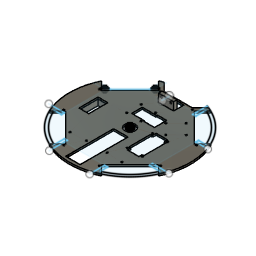
全国オフェンス上面v3 v13 (Autodesk Fusion 360 design; units mm, degrees)
Autodesk Fusion 360 part; units mm, degrees
sketch "スケッチ1" plane through (0, 0, 0) normal (0, 0, 1) x (1, 0, 0)
sketch "スケッチ2" plane through (0, 0, 0) normal (0, 0, 1) x (1, 0, 0)
  line L0 (105, 0) -> (105, 35)
  line L1 (105, 35) -> (98.9949, 35)
  line L2 (98.9949, 35) -> (78.9949, 35)
  line L3 (78.9949, 35) -> (105, 35)
  line L4 (105, 35) -> (105, -35)
  line L5 (105, -35) -> (78.9949, -35)
  line L6 (78.9949, -35) -> (78.9949, 35)
  line L7 (0, 105) -> (35, 105)
  line L8 (35, 105) -> (-35, 105)
  line L9 (-35, 105) -> (-35, 78.995)
  line L10 (-35, 78.995) -> (35, 78.995)
  line L11 (35, 78.995) -> (35, 105)
  line L12 (-105, 0) -> (-105, -35)
  line L13 (-105, -35) -> (-78.995, -35)
  line L14 (-78.995, -35) -> (-78.995, 34.9927)
  line L15 (-78.995, 34.9927) -> (-105, 34.9927)
  line L16 (-105, 34.9927) -> (-105, -35)
  line L17 (0, -105) -> (35, -105)
  line L18 (35, -105) -> (-35, -105)
  line L19 (-35, -105) -> (-35, -78.995)
  line L20 (-35, -78.995) -> (35, -78.995)
  line L21 (35, -78.995) -> (35, -105)
  arc A0 (-98.9949, -35) -> (-35, -98.9949) centre (0, 0) ccw
  arc A1 (35, -98.9949) -> (98.9949, -35) centre (0, 0) ccw
  arc A2 (98.9949, 35) -> (35, 98.9949) centre (0, 0) ccw
  arc A3 (-35, 98.9949) -> (-98.9975, 34.9927) centre (0, 0) ccw
  line L22 (-35, 98.9949) -> (-42, 98.9949)
  line L23 (-42, 98.9949) -> (-42, 96.2341)
  line L24 (-42, 96.2341) -> (-42, 76.2341)
  line L25 (-98.9975, 34.9927) -> (-98.9975, 42)
  line L26 (-98.9975, 42) -> (-96.2341, 42)
  line L27 (-96.2341, 42) -> (-76.2341, 42)
  line L28 (-76.2341, 42) -> (-42, 76.2341)
  dimension "d2" = 35
  dimension "d3" = 20
  dimension "d4" = 70
  dimension "d5" = 26.005
  dimension "d6" = 26.005
  dimension "d7" = 70
  dimension "d8" = 26.005
  dimension "d9" = 20
  dimension "d10" = 20
  constraint vertical L0
  constraint perpendicular L0 L1
  constraint perpendicular L0 L2
  constraint horizontal L3
  constraint vertical L4
  constraint horizontal L5
  constraint vertical L6
  constraint horizontal L7
  constraint horizontal L8
  constraint vertical L9
  constraint horizontal L10
  constraint vertical L11
  constraint vertical L12
  constraint horizontal L13
  constraint vertical L14
  constraint horizontal L15
  constraint vertical L16
  constraint horizontal L17
  constraint horizontal L18
  constraint vertical L19
  constraint horizontal L20
  constraint vertical L21
  constraint coincident L13 A0.start
  constraint coincident L19 A0.end
  constraint coincident L5 A1.end
  constraint coincident L21 A1.start
  constraint coincident L11 A2.end
  constraint coincident A0.centre A1.centre
  constraint coincident L15 A3.end
  constraint coincident L9 A3.start
  constraint perpendicular L9 L22
  constraint coincident A3 L23.end
  constraint perpendicular L22 L23
  constraint perpendicular L22 L24
  constraint perpendicular L15 L25
  constraint coincident A3 L26.end
  constraint perpendicular L25 L26
  constraint parallel L26 L27
  measures "d2" distance of L0.start L0.end
  measures "d3" distance of L1.end L2.end
  measures "d4" distance of L7.end L8.end
  measures "d5" distance of L7.end L10.end
  measures "d6" distance of L12.end L13.end
  measures "d7" distance of L17.end L18.end
  measures "d8" distance of L17.end L20.end
  measures "d9" distance of L23.end L24.end
  measures "d10" distance of L26.end L27.end
sketch "スケッチ3" plane through (0, 0, 0) normal (0, 0, 1) x (1, 0, 0)
  line L0 (-79, 35) -> (-74, 35)
  line L1 (-76.5, 35) -> (-76.5, 37.5)
  line L2 (-35, 79) -> (-35, 74)
  line L3 (-35, 74) -> (-35, 75)
  line L4 (-35, 76.5) -> (-37.5, 76.5)
  circle A0 centre (-37.5, 76.5) radius 1.5
  circle A1 centre (-76.5, 37.5) radius 1.5
  dimension "d11" = 3
  dimension "d12" = 3
  constraint horizontal L0
  constraint midpoint L0 L1.start
  constraint perpendicular L0 L1
  constraint vertical L2
  constraint coincident L2 L3.end
  constraint midpoint L2 L4.start
  constraint perpendicular L2 L4
  constraint coincident L4.end A0.centre
  constraint coincident L1.end A1.centre
  measures "d11" diameter of A0
  measures "d12" diameter of A1
extrude "押し出し1" add sketch "スケッチ2" along normal blind 3 contours L2 L3 L5 L6 L9 L10 L11 L13 L14 L15 L19 L20 L21 A0 A1 A2 A3 L24 L27 L28
extrude "押し出し2" cut sketch "スケッチ3" along normal blind 3
sketch "スケッチ4" plane through (0, 0, 0) normal (0, 0, 1) x (1, 0, 0)
  line L0 (79, 35) -> (74, 35)
  line L1 (74, 35) -> (74, 40)
  circle A0 centre (76.5, 37.5) radius 1.5
  line L2 (35, 79) -> (35, 74)
  line L3 (35, 74) -> (40, 74)
  circle A1 centre (37.5, 76.5) radius 1.5
  constraint horizontal L0
  constraint perpendicular L0 L1
  constraint vertical L2
  constraint perpendicular L2 L3
sketch "スケッチ5" plane through (0, 0, 3) normal (0, 0, 1) x (-1, 0, 0)
  circle A0 centre (76.5, -37.5) radius 1.5
  circle A1 centre (37.5, -76.5) radius 1.5
  arc A2 (96.2341, -42) -> (98.9975, -34.9927) centre (0, 0) ccw
  line L0 (98.9975, -34.9927) -> (78.995, -34.9927)
  line L1 (78.995, -34.9927) -> (78.995, 35)
  line L2 (78.995, 35) -> (98.9949, 35)
  arc A3 (98.9949, 35) -> (35, 98.9949) centre (0, 0) ccw
  line L3 (35, 98.9949) -> (35, 78.995)
  line L4 (35, 78.995) -> (-35, 78.995)
  line L5 (-35, 78.995) -> (-35, 98.9949)
  arc A4 (-35, 98.9949) -> (-98.9949, 35) centre (0, 0) ccw
  line L6 (-98.9949, 35) -> (-78.9949, 35)
  line L7 (-78.9949, 35) -> (-78.9949, -35)
  line L8 (-78.9949, -35) -> (-98.9949, -35)
  arc A5 (-98.9949, -35) -> (-35, -98.9949) centre (0, 0) ccw
  line L9 (-35, -98.9949) -> (-35, -78.995)
  line L10 (-35, -78.995) -> (35, -78.995)
  line L11 (35, -78.995) -> (35, -98.9949)
  arc A6 (35, -98.9949) -> (42, -96.2341) centre (0, 0) ccw
  line L12 (42, -96.2341) -> (42, -76.2341)
  line L13 (42, -76.2341) -> (76.2341, -42)
  line L14 (76.2341, -42) -> (96.2341, -42)
  line L15 (78.995, -34.9927) -> (78.995, -40)
  line L16 (78.995, -40) -> (74, -40)
  line L17 (35, -78.995) -> (40, -78.995)
  line L18 (40, -78.995) -> (40, -74)
  line L19 (40, -74) -> (74, -40)
  constraint coincident L0.end L1.start
  constraint perpendicular L0 L15
  constraint perpendicular L15 L16
  constraint coincident L10.end L11.start
  constraint perpendicular L11 L17
  constraint perpendicular L10 L18
sketch "スケッチ6" plane through (0, 0, 3) normal (0, 0, 1) x (-1, 0, 0)
  line L0 (-35, -79) -> (-35, -74)
  line L1 (-35, -74) -> (-40, -74)
  arc A0 (-91.6515, -40) -> (-40, -91.6515) centre (0, 0) ccw
  line L2 (-79, -35) -> (-100, -35)
  line L3 (-79, -35) -> (-79, -40)
  arc A1 (-98.9949, -35) -> (-34.9984, -98.9955) centre (0, 0) ccw
  line L4 (-34.9984, -98.9955) -> (-35, -79)
  line L5 (-40, -74) -> (-40, -91.6515)
  line L6 (-91.6515, -40) -> (-79, -40)
  line L7 (-79, 35) -> (-74, 35)
  line L8 (-74, 35) -> (-74, 40)
  line L9 (-79, 35) -> (-102.5239, 35)
  line L10 (-35, 79) -> (-40, 79)
  line L11 (-35, 79) -> (-35, 105)
  arc A2 (-35, 98.9949) -> (-98.9949, 35) centre (0, 0) ccw
  arc A3 (-40, 91.6515) -> (-91.6515, 40) centre (0, 0) ccw
  line L12 (-40, 79) -> (-40, 91.6515)
  line L13 (-74, 40) -> (-91.6515, 40)
  line L14 (35, 79) -> (35, 74)
  line L15 (35, 74) -> (40, 74)
  line L16 (35, 79) -> (35, 105)
  line L17 (79, 35) -> (79, 40)
  line L18 (79, 35) -> (106, 35)
  arc A4 (98.9949, 35) -> (35, 98.9949) centre (0, 0) ccw
  arc A5 (91.6515, 40) -> (40, 91.6515) centre (0, 0) ccw
  line L19 (91.6515, 40) -> (79, 40)
  line L20 (40, 74) -> (40, 91.6515)
  dimension "d17" = 100
  dimension "d18" = 105
  dimension "d19" = 105
  dimension "d20" = 100
  dimension "d21" = 105
  dimension "d22" = 100
  constraint vertical L0
  constraint perpendicular L0 L1
  constraint coincident A0.centre A1.centre
  constraint perpendicular L2 L3
  constraint coincident L2 A1.start
  constraint perpendicular L1 L5
  constraint perpendicular L3 L6
  constraint horizontal L7
  constraint perpendicular L7 L8
  constraint parallel L7 L9
  constraint horizontal L10
  constraint perpendicular L10 L11
  constraint coincident L11 A2.start
  constraint coincident L9 A2.end
  constraint perpendicular L10 L12
  constraint perpendicular L8 L13
  constraint vertical L14
  constraint perpendicular L14 L15
  constraint parallel L14 L16
  constraint vertical L17
  constraint perpendicular L17 L18
  constraint coincident L18 A4.start
  constraint coincident L16 A4.end
  constraint perpendicular L17 L19
  constraint perpendicular L15 L20
  measures "d17" radius of A0
  measures "d18" radius of A1
  measures "d19" radius of A2
  measures "d20" radius of A3
  measures "d21" radius of A4
  measures "d22" radius of A5
sketch "スケッチ7" plane through (0, 0, 3) normal (0, 0, 1) x (-1, 0, 0)
  line L0 (79, 35) -> (74, 35)
  line L1 (76.5, 35) -> (76.5, 37.5)
  line L2 (37.5, 74) -> (37.5, 76.5)
  line L3 (-37.5, 79) -> (-37.5, 76.5)
  line L4 (-74, 37.5) -> (-76.5, 37.5)
  circle A0 centre (-76.5, -37.5) radius 1.5
  circle A1 centre (-37.5, -76.5) radius 1.5
  circle A2 centre (-76.5, 37.5) radius 1.5
  circle A3 centre (-37.5, 76.5) radius 1.5
  circle A4 centre (37.5, 76.5) radius 1.5
  circle A5 centre (76.5, 37.5) radius 1.5
  dimension "d23" = 2.5
  dimension "d24" = 3
  dimension "d25" = 3
  constraint horizontal L0
  constraint midpoint L0 L1.start
  constraint perpendicular L0 L1
  constraint vertical L2
  constraint vertical L3
  constraint horizontal L4
  constraint coincident L4.end A2.centre
  constraint coincident L3.end A3.centre
  constraint coincident L2.end A4.centre
  constraint coincident L1.end A5.centre
  measures "d23" distance of L1.start L1.end
  measures "d24" diameter of A2
  measures "d25" diameter of A5
extrude "押し出し3" cut sketch "スケッチ7" against normal blind 3
sketch "スケッチ8" plane through (0, 0, 3) normal (0, 0, 1) x (-1, 0, 0)
  line L0 (-68, 68) -> (-59.1612, 76.8388)
  line L1 (-68, 68) -> (-76.8388, 59.1612)
  line L2 (-76.8388, 59.1612) -> (-20.9774, 3.2997)
  line L3 (-20.9774, 3.2997) -> (-3.2997, 20.9774)
  line L4 (-3.2997, 20.9774) -> (-59.1612, 76.8388)
  line L5 (-76.8388, 59.1612) -> (-80.7279, 55.2721)
  line L6 (-80.7279, 55.2721) -> (-55.2721, 29.8162)
  line L7 (-55.2721, 29.8162) -> (-51.383, 33.7053)
  line L8 (-51.7365, 26.2807) -> (-47.8475, 30.1698)
  arc A0 (-55.2721, 29.8162) -> (-51.7365, 26.2807) centre (-53.5043, 28.0485) ccw
  circle A1 centre (-53.5043, 28.0485) radius 1.5
  line L9 (-53.5043, 28.0485) -> (-28.0485, 53.5043)
  circle A2 centre (-28.0485, 53.5043) radius 1.5
  dimension "d28" = 12.5
  dimension "d29" = 12.5
  dimension "d30" = 79
  dimension "d31" = 25
  dimension "d33" = 5.5
  dimension "d34" = 36
  dimension "d35" = 5
  dimension "d36" = 3
  dimension "d37" = 36
  dimension "d38" = 3
  constraint perpendicular L1 L2
  constraint perpendicular L2 L5
  constraint perpendicular L5 L6
  constraint coincident L2 L7.end
  constraint perpendicular L2 L7
  constraint coincident L2 L8.end
  constraint perpendicular L2 L8
  constraint concentric A0 A1
  constraint coincident A0.centre A1.centre
  constraint perpendicular L4 L9
  constraint coincident L9.end A2.centre
  measures "d28" distance of L0.start L0.end
  measures "d29" distance of L0.start L1.end
  measures "d30" distance of L1.end L2.end
  measures "d31" distance of L2.end L3.end
  measures "d33" distance of L1.end L5.end
  measures "d34" distance of L5.end L6.end
  measures "d35" distance of L6.end L8.start
  measures "d36" diameter of A1
  measures "d37" distance of A0.centre L9.end
  measures "d38" diameter of A2
extrude "押し出し4" cut sketch "スケッチ8" against normal blind 3 contours A1 | A2
sketch "スケッチ9" plane through (0, 0, 3) normal (0, 0, 1) x (-1, 0, 0)
  line L0 (-53.5, 28) -> (-81.4307, 55.9307)
  arc A0 (-55.2678, 29.7678) -> (-51.7322, 26.2322) centre (-53.5, 28) ccw
  line L1 (-55.2678, 29.7678) -> (-51.3787, 33.6569)
  line L2 (-81.4307, 55.9307) -> (-77.5416, 59.8198)
  line L3 (-77.5416, 59.8198) -> (-21.6802, 3.9584)
  line L4 (-21.6802, 3.9584) -> (-4.0025, 21.636)
  line L5 (-4.0025, 21.636) -> (-59.864, 77.4975)
  line L6 (-59.864, 77.4975) -> (-77.5416, 59.8198)
  dimension "d43" = 39.5
  dimension "d44" = 2.5
  dimension "d45" = 5.5
  dimension "d46" = 5.5
  dimension "d47" = 79
  dimension "d48" = 25
  dimension "d49" = 79
  constraint coincident L0.start A0.centre
  constraint perpendicular L0 L1
  constraint perpendicular L0 L2
  constraint perpendicular L1 L3
  constraint perpendicular L4 L5
  constraint perpendicular L3 L6
  measures "d43" distance of L0.start L0.end
  measures "d44" radius of A0
  measures "d45" distance of A0.start L1.end
  measures "d46" distance of L0.end L2.end
  measures "d47" distance of L2.end L3.end
  measures "d48" distance of L3.end L4.end
  measures "d49" distance of L4.end L5.end
extrude "押し出し5" cut sketch "スケッチ9" against normal blind 90 contours L3 L4 L5 L6
sketch "スケッチ10" plane through (0, 0, 3) normal (0, 0, 1) x (-1, 0, 0)
sketch "スケッチ11" plane through (0, 0, 0) normal (0, 0, 1) x (1, 0, 0)
  line L0 (61.7193, 15.0503) -> (30.6066, 46.163)
  circle A0 centre (43.3345, -3.3345) radius 1.5
  circle A1 centre (61.7193, 15.0503) radius 1.5
  circle A2 centre (12.2218, 27.7782) radius 1.5
  circle A3 centre (30.6066, 46.163) radius 1.5
  line L1 (43.3345, -3.3345) -> (12.2218, 27.7782)
  line L2 (27.7782, 12.2218) -> (21.4142, 5.8579)
  line L3 (45.4558, -5.4558) -> (44.0416, -6.8701)
  line L4 (44.0416, -6.8701) -> (8.6863, 28.4853)
  line L5 (44.0416, -6.8701) -> (65.2548, 14.3431)
  line L6 (65.2548, 14.3431) -> (29.8995, 49.6985)
  line L7 (29.8995, 49.6985) -> (8.6863, 28.4853)
  line L8 (29.8995, 49.6985) -> (34.1421, 45.4558)
  line L9 (22.8284, 34.1421) -> (41.9203, 15.0503)
  circle A4 centre (22.8284, 34.1421) radius 1.5
  circle A5 centre (41.9203, 15.0503) radius 1.5
  line L10 (34.1421, 45.4558) -> (30.6066, 41.9203)
  line L11 (30.6066, 41.9203) -> (26.364, 46.163)
  line L12 (8.6863, 28.4853) -> (12.9289, 24.2426)
  line L13 (12.9289, 24.2426) -> (16.4645, 27.7782)
  line L14 (16.4645, 27.7782) -> (12.2218, 32.0208)
  line L15 (44.0416, -6.8701) -> (39.799, -2.6274)
  line L16 (44.0416, -6.8701) -> (47.5772, -3.3345)
  line L17 (47.5772, -3.3345) -> (43.3345, 0.9081)
  line L18 (39.799, -2.6274) -> (43.3345, 0.9081)
  line L19 (65.2548, 14.3431) -> (61.0122, 18.5858)
  line L20 (61.0122, 18.5858) -> (57.4767, 15.0503)
  line L21 (57.4767, 15.0503) -> (61.7193, 10.8076)
  dimension "d54" = 26
  dimension "d55" = 26
  dimension "d56" = 3
  dimension "d57" = 3
  dimension "d58" = 3
  dimension "d59" = 3
  dimension "d60" = 3
  dimension "d61" = 2
  dimension "d62" = 50
  dimension "d63" = 30
  dimension "d64" = 50
  dimension "d65" = 6
  dimension "d66" = 16
  dimension "d67" = 27
  dimension "d68" = 3
  dimension "d69" = 3
  dimension "d70" = 5
  dimension "d71" = 6
  dimension "d72" = 5
  dimension "d73" = 6
  dimension "d74" = 5
  dimension "d75" = 6
  dimension "d76" = 6
  dimension "d77" = 5
  constraint coincident L0.start A1.centre
  constraint coincident L0.end A3.centre
  constraint coincident A0.centre L1.start
  constraint coincident A2.centre L1.end
  constraint midpoint L1 L2.start
  constraint perpendicular L1 L2
  constraint perpendicular L2 L4
  constraint perpendicular L4 L5
  constraint perpendicular L5 L6
  constraint perpendicular L7 L8
  constraint coincident L9.start A4.centre
  constraint coincident L9.end A5.centre
  constraint perpendicular L0 L10
  constraint coincident L7 L11.end
  constraint perpendicular L7 L11
  constraint perpendicular L7 L12
  constraint perpendicular L1 L13
  constraint coincident L7 L14.end
  constraint perpendicular L7 L14
  constraint perpendicular L3 L15
  constraint perpendicular L15 L16
  constraint perpendicular L5 L17
  constraint perpendicular L17 L18
  constraint perpendicular L5 L19
  constraint perpendicular L0 L20
  constraint coincident L5 L21.end
  constraint perpendicular L5 L21
  measures "d54" distance of L0.end A2.centre
  measures "d55" distance of L0.start A0.centre
  measures "d56" diameter of A0
  measures "d57" diameter of A1
  measures "d58" diameter of A2
  measures "d59" diameter of A3
  measures "d60" distance of A0.centre L3.start
  measures "d61" distance of L3.start L3.end
  measures "d62" distance of L3.end L4.end
  measures "d63" distance of L3.end L5.end
  measures "d64" distance of L5.end L6.end
  measures "d65" distance of L6.end L8.end
  measures "d66" distance of L8.end L9.start
  measures "d67" distance of L9.start L9.end
  measures "d68" diameter of A4
  measures "d69" diameter of A5
  measures "d70" distance of L8.end L10.end
  measures "d71" distance of L4.end L12.end
  measures "d72" distance of L12.end L13.end
  measures "d73" distance of L3.end L15.end
  measures "d74" distance of L3.end L16.end
  measures "d75" distance of L16.end L17.end
  measures "d76" distance of L5.end L19.end
  measures "d77" distance of L19.end L20.end
extrude "押し出し6" cut sketch "スケッチ11" along normal blind 4 contours L0 L1 L5 L7 L10 L11 L13 L14 L17 L18 L20 L21 | A0 | A1 | A2 | A3 | A4 | A5
sketch "スケッチ12" plane through (0, 0, 3) normal (0, 0, 1) x (-1, 0, 0)
  line L0 (40, 40) -> (50.6066, 29.3934)
  line L1 (50.6066, 29.3934) -> (61.2132, 40)
  line L2 (61.2132, 40) -> (50.6066, 50.6066)
  line L3 (50.6066, 50.6066) -> (40, 61.2132)
  line L4 (40, 61.2132) -> (29.3934, 50.6066)
  line L5 (40, 40) -> (29.3934, 50.6066)
  dimension "d80" = 15
  dimension "d81" = 15
  dimension "d82" = 15
  dimension "d83" = 15
  dimension "d84" = 15
  constraint perpendicular L0 L1
  constraint perpendicular L3 L4
  measures "d80" distance of L0.start L0.end
  measures "d81" distance of L0.end L1.end
  measures "d82" distance of L1.end L2.end
  measures "d83" distance of L2.end L3.end
  measures "d84" distance of L3.end L4.end
extrude "押し出し7" cut sketch "スケッチ12" against normal blind 5
sketch "スケッチ13" plane through (0, 0, 0) normal (0, 0, 1) x (1, 0, 0)
  circle A0 centre (76.5, -37.5) radius 1.5
  circle A1 centre (37.5, -76.5) radius 1.5
  circle A2 centre (-37.5, -76.5) radius 1.5
  circle A3 centre (-76.5, -37.5) radius 1.5
  circle A4 centre (37.5, 76.5) radius 1.5
  circle A5 centre (76.5, 37.5) radius 1.5
extrude "押し出し8" add sketch "スケッチ4" sketch "スケッチ13" along normal blind 3 of sketch 2 contours A0 | A1 | A2 | A3
sketch "スケッチ14" plane through (0, 0, 0) normal (0, 0, 1) x (1, 0, 0)
  line L0 (79, -35) -> (79, -40)
  line L1 (79, -37.5) -> (81.5, -37.5)
  line L2 (40, -79) -> (35, -79)
  line L3 (37.5, -79) -> (37.5, -81.5)
  line L4 (-35, -79) -> (-40, -79)
  line L5 (-37.5, -79) -> (-37.5, -81.5)
  line L6 (-79, -35) -> (-79, -37.5)
  line L7 (-79, -37.5) -> (-81.5, -37.5)
  line L8 (79, 35) -> (79, 40)
  line L9 (79, 37.5) -> (81.5, 37.5)
  line L10 (35, 79) -> (40, 79)
  line L11 (37.5, 79) -> (37.5, 81.5)
  circle A0 centre (37.5, 81.5) radius 1.5
  circle A1 centre (81.5, 37.5) radius 1.5
  circle A2 centre (81.5, -37.5) radius 1.5
  circle A3 centre (37.5, -81.5) radius 1.5
  circle A4 centre (-37.5, -81.5) radius 1.5
  circle A5 centre (-81.5, -37.5) radius 1.5
  dimension "d89" = 2.5
  dimension "d90" = 2.5
  dimension "d91" = 2.5
  dimension "d92" = 2.5
  dimension "d93" = 2.5
  dimension "d94" = 2.5
  dimension "d95" = 2.5
  dimension "d96" = 3
  dimension "d97" = 3
  dimension "d98" = 3
  dimension "d99" = 3
  dimension "d100" = 3
  dimension "d101" = 3
  constraint vertical L0
  constraint midpoint L0 L1.start
  constraint perpendicular L0 L1
  constraint horizontal L2
  constraint midpoint L2 L3.start
  constraint perpendicular L2 L3
  constraint horizontal L4
  constraint midpoint L4 L5.start
  constraint perpendicular L4 L5
  constraint vertical L6
  constraint perpendicular L6 L7
  constraint vertical L8
  constraint midpoint L8 L9.start
  constraint perpendicular L8 L9
  constraint horizontal L10
  constraint midpoint L10 L11.start
  constraint perpendicular L10 L11
  constraint coincident L11.end A0.centre
  constraint coincident L9.end A1.centre
  constraint coincident L1.end A2.centre
  constraint coincident L3.end A3.centre
  constraint coincident L5.end A4.centre
  constraint coincident L7.end A5.centre
  measures "d89" distance of L1.start L1.end
  measures "d90" distance of L3.start L3.end
  measures "d91" distance of L5.start L5.end
  measures "d92" distance of L6.start L6.end
  measures "d93" distance of L6.end L7.end
  measures "d94" distance of L9.start L9.end
  measures "d95" distance of L11.start L11.end
  measures "d96" diameter of A0
  measures "d97" diameter of A1
  measures "d98" diameter of A2
  measures "d99" diameter of A3
  measures "d100" diameter of A4
  measures "d101" diameter of A5
extrude "押し出し9" cut sketch "スケッチ14" along normal blind 3
sketch "スケッチ15" plane through (0, 0, 0) normal (0, 0, 1) x (1, 0, 0)
  line L0 (12.8427, -12.8427) -> (11.3577, -11.3577)
  line L1 (11.3577, -11.3577) -> (2.5189, -20.1966)
  line L2 (2.5189, -20.1966) -> (5.3081, -22.9858)
  line L3 (11.3577, -11.3577) -> (20.1966, -2.5189)
  line L4 (20.1966, -2.5189) -> (25.4149, -7.7372)
  line L5 (25.4149, -7.7372) -> (5.3081, -22.9858)
  dimension "d104" = 2.1
  dimension "d105" = 12.5
  dimension "d106" = 12.5
  constraint perpendicular L1 L2
  constraint perpendicular L3 L4
  measures "d104" distance of L0.start L0.end
  measures "d105" distance of L0.end L1.end
  measures "d106" distance of L0.end L3.end
extrude "押し出し10" cut sketch "スケッチ15" along normal blind 3
sketch "スケッチ16" plane through (0, 0, 0) normal (0, 0, 1) x (1, 0, 0)
  line L0 (-57, 57) -> (-47.8076, 66.1924)
  line L1 (-57, 57) -> (-66.1924, 47.8076)
  line L2 (-66.1924, 47.8076) -> (-59.1213, 40.7365)
  line L3 (-59.1213, 40.7365) -> (-40.7365, 59.1213)
  line L4 (-40.7365, 59.1213) -> (-47.8076, 66.1924)
  dimension "d109" = 13
  dimension "d110" = 13
  dimension "d111" = 10
  dimension "d112" = 26
  constraint perpendicular L1 L2
  measures "d109" distance of L0.start L0.end
  measures "d110" distance of L0.start L1.end
  measures "d111" distance of L1.end L2.end
  measures "d112" distance of L2.end L3.end
extrude "押し出し11" cut sketch "スケッチ16" along normal blind 3
sketch "スケッチ17" plane through (0, 0, 0) normal (0, 0, 1) x (1, 0, 0)
  circle A0 centre (0, 0) radius 9.321
  line L0 (-40, -40) -> (-52.7279, -27.2721)
  line L1 (-52.7279, -27.2721) -> (-64.7487, -39.2929)
  line L2 (-64.7487, -39.2929) -> (-41.4142, -62.6274)
  line L3 (-41.4142, -62.6274) -> (-29.3934, -50.6066)
  line L4 (-40, -40) -> (-29.3934, -50.6066)
  dimension "d115" = 18
  dimension "d116" = 17
  dimension "d117" = 33
  dimension "d118" = 17
  constraint coincident A0.centre origin
  constraint perpendicular L0 L1
  constraint perpendicular L2 L3
  measures "d115" distance of L0.start L0.end
  measures "d116" distance of L0.end L1.end
  measures "d117" distance of L1.end L2.end
  measures "d118" distance of L2.end L3.end
extrude "押し出し12" cut sketch "スケッチ17" along normal blind 3
sketch "スケッチ18" plane through (0, 0, 3) normal (0, 0, 1) x (-1, 0, 0)
  line L0 (15, -15) -> (0, -30)
  line L1 (0, -30) -> (15, -45)
  line L2 (15, -45) -> (45, -15)
  line L3 (45, -15) -> (30, 0)
  line L4 (30, 0) -> (15, -15)
  constraint perpendicular L0 L1
  constraint perpendicular L2 L3
extrude "押し出し13" cut sketch "スケッチ18" against normal blind 3
sketch "スケッチ19" plane through (0, 0, 0) normal (0, 0, 1) x (1, 0, 0)
  line L0 (0, 0) -> (125, -125)
  line L1 (-9.1, 78.995) -> (15.9, 78.995)
  line L2 (15.9, 43.995) -> (-9.1, 43.995)
  circle A0 centre (-9.1, 43.995) radius 1.5
  circle A1 centre (15.9, 43.995) radius 1.5
  line L3 (15.9, 43.995) -> (-9.1, 43.995)
  line L4 (-9.1, 68.995) -> (15.9, 68.995)
  circle A2 centre (-9.1, 68.995) radius 1.5
  circle A3 centre (15.9, 68.995) radius 1.5
  dimension "d123" = 25
  dimension "d124" = 35
  dimension "d125" = 3
  dimension "d126" = 3
  dimension "d127" = 25
  dimension "d128" = 25
  dimension "d129" = 3
  dimension "d130" = 3
  constraint coincident L0.start origin
  constraint horizontal L1
  constraint horizontal L2
  constraint coincident L2.end A0.centre
  constraint coincident L2.start A1.centre
  constraint horizontal L3
  constraint horizontal L4
  constraint coincident L4.start A2.centre
  constraint coincident L4.end A3.centre
  measures "d123" distance of L1.start L1.end
  measures "d124" distance of L1.start L2.end
  measures "d125" diameter of A0
  measures "d126" diameter of A1
  measures "d127" distance of L2.start L2.end
  measures "d128" distance of L2.start L4.end
  measures "d129" diameter of A2
  measures "d130" diameter of A3
extrude "押し出し14" cut sketch "スケッチ19" along normal blind 20
sketch "スケッチ20" plane through (0, 0, 0) normal (0, 0, 1) x (1, 0, 0)
  line L0 (0, 0) -> (100, -100)
  line L1 (41.809, -41.809) -> (73.6288, -9.9892)
  line L2 (41.809, -41.809) -> (9.9892, -73.6288)
  circle A0 centre (73.6288, -9.9892) radius 1.5
  circle A1 centre (9.9892, -73.6288) radius 1.5
  dimension "d133" = 45
  dimension "d134" = 45
  dimension "d135" = 3
  dimension "d136" = 3
  constraint coincident L0.start origin
  constraint coincident L0 L1.start
  constraint perpendicular L0 L1
  constraint perpendicular L0 L2
  constraint coincident L1.end A0.centre
  constraint coincident L2.end A1.centre
  measures "d133" distance of L1.start L1.end
  measures "d134" distance of L1.start L2.end
  measures "d135" diameter of A0
  measures "d136" diameter of A1
extrude "押し出し15" cut sketch "スケッチ20" along normal blind 3
sketch "スケッチ21" plane through (0, 0, 0) normal (0, 0, 1) x (1, 0, 0)
  line L0 (68, -68) -> (76.8388, -59.1612)
  line L1 (76.8388, -59.1612) -> (78.9602, -61.2825)
  line L2 (78.9602, -61.2825) -> (61.2825, -78.9602)
  line L3 (61.2825, -78.9602) -> (58.0094, -75.687)
  line L4 (58.0094, -75.687) -> (68, -68)
  dimension "d139" = 12.5
  dimension "d140" = 3
  dimension "d141" = 25
  constraint perpendicular L0 L1
  constraint perpendicular L2 L3
  measures "d139" distance of L0.start L0.end
  measures "d140" distance of L0.end L1.end
  measures "d141" distance of L1.end L2.end
extrude "押し出し16" cut sketch "スケッチ21" along normal blind 30
sketch "スケッチ22" plane through (0, 0, 0) normal (0, 0, 1) x (1, 0, 0)
sketch "スケッチ23" plane through (0, 0, 0) normal (0, 0, 1) x (1, 0, 0)
  line L0 (-30, 30) -> (-15, 15)
  circle A0 centre (-13.6612, 13.6612) radius 1.5
  line L1 (-22.5, 22.5) -> (-31.3388, 31.3388)
  line L2 (-15, 15) -> (-16, 16)
  line L3 (-15, 15) -> (-17, 17)
  circle A1 centre (-31.3388, 31.3388) radius 1.5
  circle A2 centre (-49.0165, 13.6612) radius 1.5
  circle A3 centre (-31.3388, -4.0165) radius 1.5
  line L4 (-15, 15) -> (-16, 16)
  line L5 (-16, 16) -> (-30, 2)
  line L6 (-30, 30) -> (-28.562, 28.562)
  line L7 (-28.8231, 28.8231) -> (-42.8231, 14.8231)
  line L8 (-30, 30) -> (-45, 15)
  line L9 (-45, 15) -> (-30, 0)
  line L10 (-30, 0) -> (-15, 15)
  line L11 (-30, 2) -> (-42.8231, 14.8231)
  line L12 (-16, 16) -> (-12, 20)
  line L13 (-12, 20) -> (-11, 19)
  line L14 (-11, 19) -> (-15, 15)
  line L15 (-28.8231, 28.8231) -> (-26.4875, 31.1586)
  line L16 (-26.4875, 31.1586) -> (-27.6553, 32.3264)
  line L17 (-27.6553, 32.3264) -> (-30, 30)
  dimension "d144" = 12.5
  dimension "d145" = 3
  dimension "d146" = 25
  dimension "d147" = 12.5
  dimension "d148" = 25
  dimension "d149" = 3
  dimension "d150" = 3
  dimension "d151" = 3
  constraint midpoint L0 L1.start
  constraint parallel L0 L1
  constraint coincident L0 L2.end
  constraint coincident L1.end A1.centre
  constraint perpendicular L2 L5
  constraint coincident L1 L6.end
  constraint parallel L1 L6
  constraint coincident L6 L7.start
  constraint perpendicular L5 L9
  constraint perpendicular L4 L10
  constraint perpendicular L7 L11
  constraint perpendicular L3 L12
  constraint perpendicular L12 L13
  constraint perpendicular L4 L14
  constraint perpendicular L1 L15
  constraint perpendicular L15 L16
  measures "d144" distance of L1.start A0.centre
  measures "d145" diameter of A0
  measures "d146" distance of A0.centre A3.centre
  measures "d147" distance of L1.start L1.end
  measures "d148" distance of L1.end A2.centre
  measures "d149" diameter of A1
  measures "d150" diameter of A2
  measures "d151" diameter of A3
extrude "押し出し17" cut sketch "スケッチ23" along normal blind 3 contours L0 L1 L6 L15 L16 L17 | L0 L1 L2 L3 L4 L5 L6 L7 L8 L9 L10 L11 | L0 L2 L3 L4 L12 L13 L14 | A0 | A1 | A2 | A3
sketch "スケッチ24" plane through (0, 0, 3) normal (0, 0, 1) x (-1, 0, 0)
  line L0 (15, -15) -> (13, -17)
  line L1 (13, -17) -> (14, -18)
  line L2 (14, -18) -> (30, -2)
  line L3 (30, -2) -> (43, -15)
  line L4 (43, -15) -> (26, -32)
  line L5 (26, -32) -> (27, -33)
  line L6 (27, -33) -> (45, -15)
  line L7 (45, -15) -> (30, 0)
  line L8 (30, 0) -> (13, -17)
  constraint perpendicular L0 L1
  constraint perpendicular L1 L2
  constraint perpendicular L2 L3
  constraint perpendicular L3 L4
  constraint perpendicular L4 L5
  constraint perpendicular L5 L6
  constraint perpendicular L6 L7
  constraint perpendicular L1 L8
extrude "押し出し18" add sketch "スケッチ24" against normal blind 3
move_body "移動1" bodies 1 to x (0.707107, -0.707107, 0) y (0.707107, 0.707107, 0) z (0, 0, 1) at (0, 0, -3)
sketch "スケッチ25" plane through (0, 0, 0) normal (0, 0, 1) x (1, 0, 0)
  line L0 (0, 70.61) -> (13, 70.61)
  line L1 (0, 70.61) -> (-13, 70.61)
  line L2 (-13, 70.61) -> (-13, 67.61)
  line L3 (-13, 67.61) -> (13, 67.61)
  line L4 (13, 67.61) -> (13, 70.61)
  dimension "d156" = 3
  constraint horizontal L0
  constraint parallel L0 L1
  constraint perpendicular L1 L2
  constraint perpendicular L2 L3
  constraint perpendicular L0 L4
  measures "d156" distance of L1.end L2.end
extrude "押し出し19" add sketch "スケッチ25" along normal blind 20
sketch "スケッチ26" plane through (0, 0, 0) normal (0, 1, 0) x (1, 0, 0)
  line L0 (0, 0) -> (0, -10)
  line L1 (0, -10) -> (8, -10)
  line L2 (0, -10) -> (-8, -10)
  line L3 (-13, -20) -> (13, -20)
  line L4 (13, -20) -> (13, -14)
  line L5 (13, -14) -> (-13, -14)
  line L6 (-13, -14) -> (-13, -20)
  circle A0 centre (-8, -10) radius 1.5
  circle A1 centre (8, -10) radius 1.5
  dimension "d159" = 10
  dimension "d160" = 8
  dimension "d161" = 8
  dimension "d162" = 3
  dimension "d163" = 3
  constraint coincident L0.start origin
  constraint vertical L0
  constraint perpendicular L0 L1
  constraint perpendicular L0 L2
  constraint horizontal L3
  constraint vertical L4
  constraint horizontal L5
  constraint vertical L6
  constraint coincident L2.end A0.centre
  constraint coincident L1.end A1.centre
  measures "d159" distance of L0.start L0.end
  measures "d160" distance of L0.end L1.end
  measures "d161" distance of L0.end L2.end
  measures "d162" diameter of A0
  measures "d163" diameter of A1
extrude "押し出し20" cut sketch "スケッチ26" along normal blind 90
sketch "スケッチ27" plane through (0, 0, 0) normal (0, 0, 1) x (1, 0, 0)
move_body "移動2" bodies 1 to x (1, 0, 0) y (0, 1, 0) z (0, 0, 1) at (0, 0, 3)
sketch "スケッチ28" plane through (0, 0, 0) normal (0, 0, 1) x (1, 0, 0)
  line L0 (-56.5678, 18.0011) -> (-73.569, 18.0011)
  line L1 (-73.569, 18.0011) -> (-73.569, -15.0006)
  line L2 (-73.569, -15.0006) -> (-56.5678, -15.0006)
  line L3 (-56.5678, -15.0006) -> (-56.5678, 18.0011)
  line L4 (-73.569, -15.0006) -> (-75.4815, -15.0006)
  line L5 (-75.4815, -15.0006) -> (-75.4815, -17)
  line L6 (-75.4815, -17) -> (-53.598, -17)
  line L7 (-53.598, -17) -> (-53.598, 20.7886)
  line L8 (-53.598, 20.7886) -> (-75.4815, 20.7886)
  line L9 (-75.4815, 20.7886) -> (-75.4815, -17)
  constraint horizontal L0
  constraint vertical L1
  constraint horizontal L2
  constraint vertical L3
  constraint perpendicular L1 L4
  constraint perpendicular L4 L5
  constraint horizontal L6
  constraint vertical L7
  constraint horizontal L8
  constraint vertical L9
extrude "押し出し21" add sketch "スケッチ28" against normal blind 10
extrude "押し出し22" add 1 faces at (-2.4167, 67.61, 5.9003) along direction (0, -1, 0) blind 3
extrude "押し出し23" cut 1 faces at (2.4167, 70.61, 5.9003) along direction (0, -1, 0) blind 2
sketch "スケッチ29" plane through (0, 0, 3) normal (0, 0, 1) x (-1, 0, 0)
  line L0 (-13, -68.6) -> (13, -68.6)
  line L1 (13, -68.6) -> (13, -73)
  line L2 (13, -73) -> (-13, -73)
  line L3 (-13, -73) -> (-13, -68.6)
  constraint horizontal L0
  constraint vertical L1
  constraint horizontal L2
  constraint vertical L3
extrude "押し出し24" cut sketch "スケッチ29" against normal blind 3
sketch "スケッチ30" plane through (0, 0, 3) normal (0, 0, 1) x (-1, 0, 0)
  line L0 (13, -80.6) -> (13, -68.6)
  constraint vertical L0
extrude "押し出し25" add 1 faces at (-2.4167, 64.61, 5.9003) along direction (0, -1, 0) blind 2
